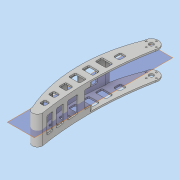
# Autodesk Inventor part: Spi_Leg_1
Saved by Autodesk Inventor 2018 (Build 220112000, 112)
## iProperties
Created: 2019-04-21
Part Number: Spi_Leg_1
Material: 일반
Document SubType Name: Modeling
Designer: khopa
Density: 1 g/cm^3
Appearance: 기본값
Author: khopa
Autodesk Inventor part; units mm, degrees
ref_plane "YZ Plane" through (0, 0, 0) normal (1, 0, 0) x (0, 1, 0)
ref_plane "XZ Plane" through (0, 0, 0) normal (0, 1, 0) x (-1, 0, 0)
ref_plane "XY Plane" through (0, 0, 0) normal (0, 0, 1) x (1, 0, 0)
sketch "스케치1" plane through (0, 0, 0) normal (0, 0, 1) x (1, 0, 0)
  circle A0 centre (0, 0) radius 8 construction
  circle A1 centre (0, 8) radius 1.2
  circle A2 centre (-8, 0) radius 1.2
  circle A3 centre (0, -8) radius 1.2
  circle A4 centre (8, 0) radius 1.2
  circle A5 centre (0, 0) radius 11
  circle A6 centre (0, 0) radius 3.5
  dimension "d0" = 16
  dimension "d1" = 2.4
  dimension "d2" = 2.4
  dimension "d3" = 2.4
  dimension "d4" = 2.4
  dimension "d5" = 22
  dimension "d6" = 7
  constraints: 7 centre point, 4 point on circle, 3 coincident
  measures "d0" diameter of A0
  measures "d1" diameter of A1
  measures "d2" diameter of A2
  measures "d3" diameter of A3
  measures "d4" diameter of A4
  measures "d5" diameter of A5
  measures "d6" diameter of A6
extrude "돌출1" add sketch "스케치1" along normal blind 2.5
sketch "스케치2" plane through (0, 0, 2.5) normal (0, 0, 1) x (1, 0, 0)
  circle A0 centre (0, 0) radius 3.5 projected
  circle A1 centre (8, 0) radius 1.2 projected
  circle A2 centre (0, -8) radius 1.2 projected
  circle A3 centre (-8, 0) radius 1.2 projected
  circle A4 centre (0, 8) radius 1.2 projected
  circle A5 centre (0, 0) radius 11 projected
  circle A6 centre (0, -180) radius 8
  arc A7 (-11, 0) -> (-8, -180) centre (202.1254, -86.4729) ccw
  arc A8 (11, 0) -> (8, -180) centre (501.2627, -98.196) ccw
  dimension "d9" = 16
  dimension "d10" = 180
  dimension "d11" = 0
  dimension "d12" = 230
  dimension "d13" = 500
  constraints: 8 point on circle, 3 centre point
  measures "d9" diameter of A6
  measures "d10" distance of A6.centre point (0, 0)
  measures "d11" horizontal distance of A6.centre point (0, 0)
  measures "d12" radius of A7
  measures "d13" radius of A8
extrude "돌출2" add sketch "스케치2" against normal blind 2.5 contours A8 A5 | A5 A8 A6 A7 | A6 A8 picked at (-6.1426, 3.5791) picked at (-2.6819, -180.0731)
ref_plane "작업 평면1" through (0, 0, -20) normal (0, 0, -1) x (-1, 0, 0)
sketch "스케치3" plane through (0, 0, 0) normal (0, 0, -1) x (-1, 0, 0)
  circle A0 centre (0, 8) radius 1.2 projected
  circle A1 centre (8, 0) radius 1.2 projected
  circle A2 centre (0, -8) radius 1.2 projected
  circle A3 centre (-8, 0) radius 1.2 projected
  circle A4 centre (0, 0) radius 3.5 projected
  arc A5 (11, 0) -> (-10.1869, -4.1505) centre (0, 0) ccw projected
  arc A6 (-8, -180) -> (-10.1869, -4.1505) centre (-501.2627, -98.196) ccw projected
  arc A7 (-8, -180) -> (8, -180) centre (0, -180) ccw projected
  arc A8 (8, -180) -> (11, 0) centre (-202.1254, -86.4729) ccw projected
  arc A9 (8.9923, -0.3723) -> (-8.2619, -3.5694) centre (0, 0) ccw
  arc A10 (-5.9981, -180.1528) -> (0.7208, -94.124) centre (-501.2627, -98.196) ccw
  arc A11 (-5.9981, -180.1528) -> (5.9869, -179.6034) centre (0, -180) ccw
  line L0 (22.9384, -50) -> (23.7506, -43.1137)
  arc A12 (5.9869, -179.6034) -> (22.9384, -50) centre (-202.1254, -86.4729) ccw
  arc A13 (9.0655, -0.552) -> (8.9923, -0.3723) centre (-202.1254, -86.4729) ccw
  line L1 (0.7208, -94.124) -> (-1.2627, -98.0632)
  dimension "d18" = 50
  dimension "d19" = 160
  constraints: 12 point on circle, 5 centre point, 4 end point, 2 other
  measures "d18" vertical distance of point (0, 0) L0.start
  measures "d19" angle of L0 L1
extrude "돌출3" add sketch "스케치3" along normal blind 40 contours A8 A7 A6 L1 A10 A11 A12 L0
mirror "미러1" about plane through (0, 0, -20) normal (0, 0, -1) of "돌출2", "돌출1"
sketch "스케치4" plane through (0, 0, 2.5) normal (0, 0, 1) x (1, 0, 0)
  arc A0 (-8, -180) -> (8, -180) centre (0, -180) ccw projected
  arc A1 (-11, 0) -> (-8, -180) centre (202.1254, -86.4729) ccw projected
  arc A2 (10.1869, -4.1505) -> (-11, 0) centre (0, 0) ccw projected
  arc A3 (10.1869, -4.1505) -> (8, -180) centre (501.2627, -98.196) ccw projected
  circle A4 centre (0, 0) radius 3.5 projected
  circle A5 centre (8, 0) radius 1.2 projected
  circle A6 centre (0, -8) radius 1.2 projected
  circle A7 centre (-8, 0) radius 1.2 projected
  circle A8 centre (0, 8) radius 1.2 projected
  line L0 (-13, -36) -> (-3.5, -36)
  line L1 (-3.5, -36) -> (-3.5, -47)
  line L2 (-3.5, -47) -> (-13, -47)
  line L3 (-13, -47) -> (-13, -36)
  line L4 (-3.5, -57) -> (-21, -57)
  line L5 (-21, -57) -> (-21, -68)
  line L6 (-21, -68) -> (-3.5, -68)
  line L7 (-3.5, -68) -> (-3.5, -57)
  line L8 (-3.5, -78) -> (-21, -78)
  line L9 (-21, -78) -> (-21, -89)
  line L10 (-21, -89) -> (-3.5, -89)
  line L11 (-3.5, -89) -> (-3.5, -78)
  line L12 (-3.5, -99) -> (-21, -99)
  line L13 (-21, -99) -> (-21, -110)
  line L14 (-21, -110) -> (-3.5, -110)
  line L15 (-3.5, -110) -> (-3.5, -99)
  line L16 (-3.5, -120) -> (-15.5, -120)
  line L17 (-15.5, -120) -> (-15.5, -131)
  line L18 (-15.5, -131) -> (-3.5, -131)
  line L19 (-3.5, -131) -> (-3.5, -120)
  line L20 (-3.5, -141) -> (-13, -141)
  line L21 (-13, -141) -> (-13, -150)
  line L22 (-13, -150) -> (-3.5, -150)
  line L23 (-3.5, -150) -> (-3.5, -141)
  line L24 (0, -160) -> (-8, -160)
  line L25 (-8, -160) -> (-8, -169)
  line L26 (0, -169) -> (0, -160)
  line L27 (-8, -169) -> (0, -169)
  dimension "d22" = 11
  dimension "d23" = 10
  dimension "d24" = 10
  dimension "d25" = 10
  dimension "d26" = 10
  dimension "d27" = 10
  dimension "d28" = 10
  dimension "d29" = 11
  dimension "d30" = 11
  dimension "d31" = 11
  dimension "d32" = 9
  dimension "d33" = 11
  dimension "d34" = 9
  dimension "d35" = 36
  dimension "d36" = 9.5
  dimension "d37" = 17.5
  dimension "d38" = 12
  dimension "d39" = 8
  dimension "d44" = 3.5
  constraints: 56 end point, 13 parallel, 8 horizontal, 8 point on line, 7 perpendicular
  measures "d22" distance of L9.end L8.end
  measures "d23" distance between parallel lines of L4 L2
  measures "d24" distance between parallel lines of L8 L6
  measures "d25" distance between parallel lines of L12 L10
  measures "d26" distance between parallel lines of L16 L14
  measures "d27" distance between parallel lines of L20 L18
  measures "d28" distance between parallel lines of L24 L22
  measures "d29" distance of L6.end L4.start
  measures "d30" distance of L14.end L12.start
  measures "d31" distance of L18.end L16.start
  measures "d32" distance of L22.end L20.start
  measures "d33" distance of L1.end L0.end
  measures "d34" distance of L26.start L24.start
  measures "d35" vertical distance of point (0, 0) L0.end
  measures "d36" distance of L0.start L0.end
  measures "d37" distance of L4.start L4.end
  measures "d38" distance of L16.start L16.end
  measures "d39" distance of L24.start L24.end
  measures "d44" distance between parallel lines of L23 L26
extrude "돌출4" cut sketch "스케치4" against normal blind 2.5 contours L0 L1 L2 L3 | L7 L6 L5 L4 | L11 L10 L9 L8 | L15 L14 L13 L12 | L19 L18 L17 L16 | L23 L22 L21 L20 | L26 L27 L25 L24
fillet "모깎기1" radius 2 14 edges at (-13, -36, 1.25) (-3.5, -36, 1.25) (-3.5, -57, 1.25) (-3.5, -68, 1.25) (-3.5, -78, 1.25) (-3.5, -89, 1.25) (-3.5, -99, 1.25) (-3.5, -110, 1.25) (-3.5, -120, 1.25) (-3.5, -131, 1.25) (-3.5, -141, 1.25) (-3.5, -150, 1.25) (0, -160, 1.25) (0, -169, 1.25)
fillet "모깎기2" radius 2 14 edges at (-13, -47, 1.25) (-21, -57, 1.25) (-21, -68, 1.25) (-21, -78, 1.25) (-21, -89, 1.25) (-21, -99, 1.25) (-21, -110, 1.25) (-15.5, -120, 1.25) (-15.5, -131, 1.25) (-13, -141, 1.25) (-13, -150, 1.25) (-8, -160, 1.25) (-8, -169, 1.25) (-3.5, -47, 1.25)
mirror "미러2" about plane through (0, 0, -20) normal (0, 0, -1) of "모깎기1", "돌출4", "모깎기2"
sketch "스케치5" plane through (0, 0, 0) normal (1, 0, 0) x (0, 1, 0)
  line L0 (24, -20) -> (-194, -20)
  line L1 (-4.1505, 0) -> (11, 0) projected
  line L2 (-63, -33) -> (-77, -33)
  line L3 (-79, -31) -> (-79, -8)
  line L4 (-77, -6) -> (-63, -6)
  line L5 (-61, -8) -> (-61, -31)
  line L6 (-91, -6) -> (-105, -6)
  line L7 (-107, -8) -> (-107, -31)
  line L8 (-105, -33) -> (-91, -33)
  line L9 (-89, -31) -> (-89, -8)
  line L10 (-120, -6) -> (-133, -6)
  line L11 (-135, -8) -> (-135, -31)
  line L12 (-133, -33) -> (-120, -33)
  line L13 (-118, -31) -> (-118, -8)
  line L14 (-144, -6) -> (-153, -6)
  line L15 (-155, -8) -> (-155, -31)
  line L16 (-153, -33) -> (-144, -33)
  line L17 (-142, -31) -> (-142, -8)
  line L18 (-163, -6) -> (-170, -6)
  line L19 (-172, -8) -> (-172, -31)
  line L20 (-170, -33) -> (-163, -33)
  line L21 (-161, -31) -> (-161, -8)
  arc A0 (-61, -8) -> (-63, -6) centre (-63, -8) ccw
  arc A1 (-63, -33) -> (-61, -31) centre (-63, -31) ccw
  arc A2 (-89, -8) -> (-91, -6) centre (-91, -8) ccw
  arc A3 (-91, -33) -> (-89, -31) centre (-91, -31) ccw
  arc A4 (-77, -6) -> (-79, -8) centre (-77, -8) ccw
  arc A5 (-79, -31) -> (-77, -33) centre (-77, -31) ccw
  arc A6 (-105, -6) -> (-107, -8) centre (-105, -8) ccw
  arc A7 (-107, -31) -> (-105, -33) centre (-105, -31) ccw
  arc A8 (-118, -8) -> (-120, -6) centre (-120, -8) ccw
  arc A9 (-133, -6) -> (-135, -8) centre (-133, -8) ccw
  arc A10 (-135, -31) -> (-133, -33) centre (-133, -31) ccw
  arc A11 (-120, -33) -> (-118, -31) centre (-120, -31) ccw
  arc A12 (-142, -8) -> (-144, -6) centre (-144, -8) ccw
  arc A13 (-153, -6) -> (-155, -8) centre (-153, -8) ccw
  arc A14 (-155, -31) -> (-153, -33) centre (-153, -31) ccw
  arc A15 (-144, -33) -> (-142, -31) centre (-144, -31) ccw
  arc A16 (-161, -8) -> (-163, -6) centre (-163, -8) ccw
  arc A17 (-170, -6) -> (-172, -8) centre (-170, -8) ccw
  arc A18 (-172, -31) -> (-170, -33) centre (-170, -31) ccw
  arc A19 (-163, -33) -> (-161, -31) centre (-163, -31) ccw
  point P0 (0, 0)
  point P1 (-89, -6)
  point P2 (-107, -33)
  point P3 (-142, -6)
  point P4 (-155, -33)
  point P5 (-161, -6)
  point P6 (-172, -33)
  dimension "d45" = 20
  dimension "d46" = 2
  dimension "d47" = 2
  constraints: 42 end point, 40 point on circle, 40 tangent, 20 centre point, 18 equal radius, 18 point on line, 10 parallel, 6 horizontal, 5 perpendicular
  measures "d45" distance between parallel lines of L1 L0
  measures "d46" radius of A0
  measures "d47" radius of A16
extrude "돌출5" cut sketch "스케치5" along normal through all both and the other way through all
